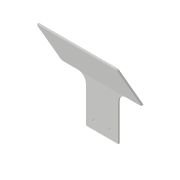
# Autodesk Inventor part: DeliveryBoxBackstop
Saved by Autodesk Inventor 2018 (Build 220112000, 112)
## iProperties
Created: 2019-02-21
Part Number: DeliveryBoxBackstop
Material: Generic
Document SubType Name: Modeling
Designer: ball
Density: 1 g/cm^3
Appearance: Default
Author: ball
Autodesk Inventor part; units mm, degrees
ref_plane "YZ Plane" through (0, 0, 0) normal (1, 0, 0) x (0, 1, 0)
ref_plane "XZ Plane" through (0, 0, 0) normal (0, 1, 0) x (-1, 0, 0)
ref_plane "XY Plane" through (0, 0, 0) normal (0, 0, 1) x (1, 0, 0)
sketch "Sketch1" plane through (0, 0, 0) normal (0, 0, 1) x (1, 0, 0)
  line L0 (0, 0) -> (50.8, 0)
  line L1 (50.8, 0) -> (50.8, 69.85)
  line L2 (50.8, 69.85) -> (0, 69.85)
  line L3 (0, 69.85) -> (0, 0)
  dimension "d0" = 50.8
  dimension "d1" = 69.85
  constraints: 8 end point, 2 parallel, 1 horizontal, 1 perpendicular
  measures "d0" distance of L2.end L1.end
  measures "d1" distance of L1.end L0.end
extrude "Extrusion1" add sketch "Sketch1" along normal blind 2.54
sketch "Sketch2" plane through (50.8, 0, 0) normal (1, 0, 0) x (0, 0, -1)
  line L0 (0, 0) -> (0, 69.85) construction
  line L1 (0, 69.85) -> (0, 139.7) construction
  line L2 (-2.54, 0) -> (-2.54, 69.85) construction
  line L3 (-2.54, 69.85) -> (-42.8679, 139.7)
  line L4 (-2.54, 69.85) -> (78.1158, 69.85) construction
  line L5 (-42.8679, 139.7) -> (-40.6682, 140.97)
  line L6 (-40.6682, 140.97) -> (0, 70.5306)
  line L7 (0, 69.85) -> (-2.54, 69.85) projected
  line L8 (0, 70.5306) -> (0, 69.85)
  dimension "d4" = 69.85
  dimension "d5" = 120
  dimension "d6" = 2.54
  constraints: 12 end point, 1 collinear, 1 equal length, 1 horizontal, 1 parallel, 1 point on line, 1 vertical
  measures "d4" distance of L0.end L1.end
  measures "d5" angle of L4 L3
  measures "d6" distance of L3.end L5.end
extrude "Extrusion2" add sketch "Sketch2" along normal blind 38.1 and the other way blind 88.9
fillet "Fillet1" radius 12.7 2 edges at (0, 69.85, 1.27) (50.8, 69.85, 1.27)
fillet "Fillet2" radius 3.175 4 edges at (88.9, 140.335, 41.7681) (-38.1, 140.335, 41.7681) (-38.1, 69.85, 1.27) (88.9, 69.85, 1.27)
sketch "Sketch3" plane through (0, 0, 2.54) normal (0, 0, 1) x (1, 0, 0)
  line L0 (0, 0) -> (50.8, 0) projected
  line L1 (0, 57.15) -> (0, 0) projected
  line L2 (50.8, 0) -> (50.8, 57.15) projected
  point P0 (12.7, 12.7)
  point P1 (38.1, 12.7)
  dimension "d13" = 12.7
  dimension "d14" = 12.7
  dimension "d15" = 12.7
  dimension "d16" = 12.7
  measures "d13" distance from line of L0 point (12.7, 12.7)
  measures "d14" distance from line of L1 point (12.7, 12.7)
  measures "d15" distance from line of L2 point (38.1, 12.7)
  measures "d16" distance from line of L0 point (38.1, 12.7)
hole "Hole1" at (12.7, 12.7, 2.54) at (38.1, 12.7, 2.54) direction (0, 0, -1) diameter 3.937 end through all
body "Solid1"
